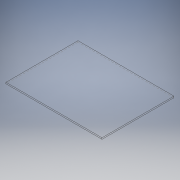
# Autodesk Inventor part: Drawer bottom
Saved by Autodesk Inventor 2016 (Build 200138000, 138)
## iProperties
Created: 2017-10-31
Part Number: Drawer bottom
Material: ABS Plastic
Document SubType Name: Modeling
Designer: mathaetaes
Density: 1.06 g/cm^3
Appearance: Smooth - White
Author: mathaetaes
Autodesk Inventor part; units mm, degrees
ref_plane "YZ Plane" through (0, 0, 0) normal (1, 0, 0) x (0, 1, 0)
ref_plane "XZ Plane" through (0, 0, 0) normal (0, 1, 0) x (-1, 0, 0)
ref_plane "XY Plane" through (0, 0, 0) normal (0, 0, 1) x (1, 0, 0)
sketch "Sketch1" plane through (0, 0, 0) normal (0, 1, 0) x (-1, 0, 0)
  line L0 (225.4564, 38.988) -> (-219.0436, 38.988)
  line L1 (-219.0436, 38.988) -> (-219.0436, -284.862)
  line L2 (-219.0436, -284.862) -> (225.4564, -284.862)
  line L3 (225.4564, -284.862) -> (225.4564, 38.988)
  point P0 (0, 0)
  dimension "d0" = 444.5
  dimension "d1" = 323.85
  constraints: 8 end point, 2 parallel, 1 horizontal, 1 perpendicular
  measures "d0" distance of L1.end L2.end
  measures "d1" distance of L0.end L1.end
extrude "Extrusion1" add sketch "Sketch1" along normal blind 6.35
body "Solid1"
